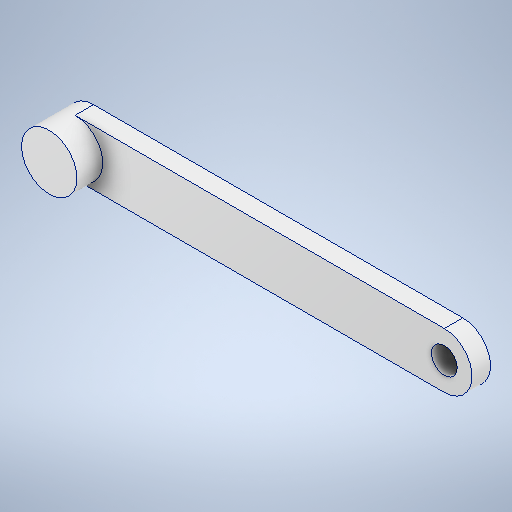
# Autodesk Inventor part: L2
Saved by Autodesk Inventor 2025 (Build 290162000, 162)
## iProperties
Created: 2023-05-06
Part Number: L2
Material: Aluminio 6061
Document SubType Name: Modeling
Designer: Miguel Ángel
Density: 2.7 g/cm^3
Appearance: Aluminio - Plano
Author: Miguel Ángel
Autodesk Inventor part; units mm, degrees
ref_plane "YZ Plane" through (0, 0, 0) normal (1, 0, 0) x (0, 1, 0)
ref_plane "XZ Plane" through (0, 0, 0) normal (0, 1, 0) x (-1, 0, 0)
ref_plane "XY Plane" through (0, 0, 0) normal (0, 0, 1) x (1, 0, 0)
sketch "Boceto1" plane through (0, 0, 0) normal (0, 0, 1) x (1, 0, 0)
  line L0 (-20.4169, 0) -> (79.5831, 0) construction
  line L1 (-20.4169, -7.5) -> (79.5831, -7.5)
  line L2 (79.5831, 7.5) -> (-20.4169, 7.5)
  arc A0 (-20.4169, 7.5) -> (-20.4169, -7.5) centre (-20.4169, 0) ccw
  arc A1 (79.5831, -7.5) -> (79.5831, 7.5) centre (79.5831, 0) ccw
  circle A2 centre (79.5831, 0) radius 3.5
  point P0 (0, 0)
  point P1 (29.5831, 0)
  dimension "d0" = 100
  dimension "d1" = 15
  dimension "d2" = 7
  constraints: 8 end point, 4 point on circle, 4 tangent, 3 centre point, 1 coincident, 1 horizontal, 1 midpoint, 1 parallel
  measures "d0" distance of L0.start L0.end
  measures "d1" diameter of A1
  measures "d2" diameter of A2
extrude "Extrusión1" add sketch "Boceto1" along normal blind 5
sketch "Boceto3" plane through (0, 0, 5) normal (0, 0, 1) x (1, 0, 0)
  line L0 (79.5831, 7.5) -> (-20.4169, 7.5) projected
  circle A0 centre (-20.4169, 0) radius 7.5
  point P0 (0, 0)
  constraints: 1 vertical alignment, 2 other
extrude "Extrusión3" add sketch "Boceto3" along normal blind 7
